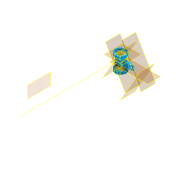
# Autodesk Inventor part: bistability_test_rack_45_0.8
Saved by Autodesk Inventor 2021 (Build 250183000, 183)
## iProperties
Created: 2021-01-14
Part Number: bistability_test_rack_45_0.8
Material: Generic
Document SubType Name: Modeling
Designer: Fierce PC
Density: 1 g/cm^3
Appearance: Default
Author: Fierce PC
Autodesk Inventor part; units mm, degrees
ref_plane "XZ Plane" through (0, 0, 0) normal (0, 1, 0) x (-1, 0, 0)
sketch "Sketch2" plane through (0, 0, 0) normal (0, 1, 0) x (-1, 0, 0)
  circle A0 centre (0, 0) radius 2
  circle A1 centre (0, 0) radius 1
  dimension "d0" = 4
  dimension "d1" = 2
  constraints: 2 centre point, 2 coincident
  measures "d0" diameter of A0
  measures "d1" diameter of A1
extrude "Extrusion1" add sketch "Sketch2" along normal blind 2 and the other way blind 2.5
sketch "Sketch3" plane through (0, 0, 0) normal (1, 0, 0) x (0, 1, 0)
  line L0 (2, -2) -> (2, 2) projected
  line L1 (-4.506, 0) -> (6.036, 0) projected
  line L2 (-2.5, 2) -> (2, 2) projected
  line L3 (-2.5, 4) -> (2, 4) projected
  arc A0 (2.1798, 2.5374) -> (2, 2) centre (2.8929, 2) ccw
  line L4 (2, 2) -> (2, 1)
  line L5 (2, 1) -> (-2.5, 1) projected
  line L6 (2.7766, 1) -> (2, 1)
  line L7 (2.7766, 1) -> (2.7766, 2)
  line L8 (2.7766, 2) -> (4.6605, 4.5)
  line L9 (2.1798, 2.5374) -> (3.6587, 4.5)
  line L10 (4.6605, 4.5) -> (3.6587, 4.5)
  point P0 (0, 0)
  dimension "d95" = 37
  dimension "d96" = 0.8
  dimension "d99" = 2.5
  constraints: 12 end point, 2 horizontal alignment, 2 point on circle, 2 point on line, 2 tangent, 1 centre point, 1 horizontal, 1 parallel, 1 perpendicular, 1 vertical, 1 other
  measures "d96" distance between parallel lines of L8 L9
  measures "d99" vertical distance of L7.end L8.end
revolve "Revolution1" add sketch "Sketch3" angle 360 about axis through (0, -10, 0) along (0, 1, 0) separate body
sketch "Sketch4" plane through (0, 0, 0) normal (0, 0, 1) x (1, 0, 0)
  line L0 (0, -0.906) -> (0, 5.436) projected
  line L1 (4.5, 4.6605) -> (-4.5, 4.6605) projected
  line L2 (4.5, 4.6605) -> (6.5, 4.6605)
  line L3 (6.5, 4.6605) -> (6.5, 3.6587)
  line L4 (6.5, 3.6587) -> (4.5, 3.6587)
  line L5 (4.5, 3.6587) -> (4.5, 4.6605)
  line L6 (2.5374, 2.1798) -> (4.5, 3.6587) projected
  line L7 (4.5, 3.6587) -> (4.5, 4.6605) projected
  point P0 (0, 0)
  dimension "d178" = 2
  constraints: 8 end point, 2 parallel, 1 coincident, 1 horizontal, 1 perpendicular
  measures "d178" distance of L1.start L2.end
revolve "Revolution2" add sketch "Sketch4" angle 360 about axis through (0, -10, 0) along (0, 1, 0) separate body
sketch "Sketch15" plane through (0, -2.5, 0) normal (0, -1, 0) x (1, 0, 0)
  circle A0 centre (0, 0) radius 2.7574 projected
  circle A1 centre (0, 0) radius 2
  dimension "d73" = 4
  constraints: 1 centre point, 1 coincident
  measures "d73" diameter of A1
extrude "Extrusion9" add sketch "Sketch15" along normal blind 0.5 contours A1 bodies 1
ref_plane "Work Plane6" through (0, 0, 0) normal (0.1736482, 0, 0.9848078) x (0, 1, 0)
ref_plane "Work Plane5" through (4.7625, 0, 0) normal (1, 0, 0) x (0, 1, 0)
sketch "Sketch21" plane through (0, 4.6605, 0) normal (0, 1, 0) x (1, 0, 0)
  arc A0 (-3.2392, 7.3149) -> (-5.022, 6.2273) centre (0, 0) ccw
  arc A1 (-3.6238, 8.1836) -> (-5.6184, 6.9668) centre (0, 0) ccw
  line L0 (-5.6184, 6.9668) -> (-5.022, 6.2273)
  line L1 (-3.2392, 7.3149) -> (-3.6238, 8.1836)
  dimension "d100" = 15
  dimension "d101" = 0.95
  constraints: 4 end point, 4 point on circle, 2 centre point, 1 coincident
  measures "d101" radial gap between concentric circles of A0 A1
extrude "Extrusion13" [suppressed]
sketch "Sketch23" plane through (-5.022, 7.0569, -6.2273) normal (-0.778413, 0, 0.6277525) x (0.6277525, 0, 0.778413)
  line L0 (-0.95, 2.3) -> (0, 2.3) projected
  line L1 (0, 0) -> (0, 2.3) projected
  line L2 (-0.95, 2.3) -> (0, 2.3)
  line L3 (0, 2.3) -> (0, 1.1)
  line L4 (0, 1.1) -> (-0.95, 1.1)
  line L5 (-0.95, 1.1) -> (-0.95, 2.3)
  line L6 (8, -14.3283) -> (8, 5.0714) projected
  point P0 (8, -7.0569)
  dimension "d105" = 1.2
  constraints: 8 end point, 2 parallel, 1 horizontal, 1 perpendicular, 1 point on line
  measures "d105" distance between parallel lines of L0 L4
revolve "Revolution3" [suppressed]
fillet "Fillet3" [suppressed]
pattern_circular "Circular Pattern5" [suppressed]
ref_plane "Work Plane8" through (4, 0, 0) normal (1, 0, 0) x (0, 1, 0)
sketch "Sketch26" plane through (4, 0, 0) normal (1, 0, 0) x (0, 1, 0)
  line L0 (-3, 2) -> (-3, -2) projected
  line L1 (0, -4) -> (-3, -4)
  line L2 (-3, -4) -> (-3, 4)
  line L3 (-3, 4) -> (0, 4)
  line L4 (0, 4) -> (0, -4)
  point P0 (0, 0)
  point P1 (0, 0)
  point P2 (-4, -3)
  dimension "d115" = 8
  dimension "d117" = 3
  constraints: 8 end point, 2 parallel, 1 coincident, 1 horizontal, 1 midpoint, 1 perpendicular, 1 point on line
  measures "d115" distance of L3.end L1.start
  measures "d117" distance of L1.start L1.end
extrude "Extrusion14" add sketch "Sketch26" against normal up to surface (4 mm away) bodies 1
pattern_circular "Circular Pattern6" count 2 over 360 about axis through (0, 4.1596, 0) along (0, -1, 0) of "Extrusion14" bodies 1
sketch "Sketch27" plane through (0, 4.6605, 0) normal (0, 1, 0) x (1, 0, 0)
  circle A0 centre (0, 0) radius 2.5374 projected
  circle A1 centre (0, 0) radius 6.5
  circle A2 centre (0, 0) radius 5.5
  dimension "d125" = 1
  dimension "d128" = 13
  constraints: 2 centre point, 2 coincident
  measures "d125" radial gap between concentric circles of A1 A2
  measures "d128" diameter of A1
extrude "Extrusion15" add sketch "Sketch27" along normal blind 2 contours A1 bodies 3
mirror "Mirror3" about plane through (0, -3, 0) normal (0, -1, 0) bodies 3 2 1
sketch "Sketch19" plane through (4.7625, 0, 0) normal (1, 0, 0) x (0, 1, 0)
  line L0 (-1, 3) -> (-7, 3)
  line L1 (-7, 3) -> (-7, 6.2171)
  line L2 (-7, 6.2171) -> (-1, 6.2171)
  line L3 (-1, 6.2171) -> (-1, 3)
  line L4 (-1, -3) -> (-7, -3)
  line L5 (-7, -3) -> (-7, -7.1834)
  line L6 (-7, -7.1834) -> (-1, -7.1834)
  line L7 (-1, -7.1834) -> (-1, -3)
  point P0 (0, 0)
  dimension "d81" = 6
  dimension "d82" = 7
  dimension "d83" = 3
  dimension "d84" = 6
  dimension "d85" = 3
  constraints: 16 end point, 4 parallel, 2 horizontal, 2 perpendicular
  measures "d81" distance of L1.end L2.end
  measures "d82" horizontal distance of L0.end point (0, 0)
  measures "d83" distance from line of point (0, 0) L0
  measures "d84" distance of L5.end L6.end
  measures "d85" distance from line of L4 point (0, 0)
extrude "Extrusion11" [suppressed]
fillet "Fillet2" radius 2 2 edges at (0, 2.7766, -2) (0, -8.7766, -2)
sketch "Sketch34" plane through (0, -6, 0) normal (0, -1, 0) x (1, 0, 0)
  circle A0 centre (0, 0) radius 1
  dimension "d160" = 2
  constraints: 1 centre point, 1 coincident
  measures "d160" diameter of A0
extrude "Extrusion20" cut sketch "Sketch34" against normal blind 1.5 bodies 1
ref_plane "Work Plane15" through (-3, 0, -5) normal (0, 1, 0) x (1, 0, 0)
sketch "Sketch36" plane through (-3, 0, -5) normal (0, 1, 0) x (1, 0, 0)
  circle A0 centre (3, -5) radius 1
  dimension "d161" = 2
  constraints: 1 centre point, 1 coincident
  measures "d161" diameter of A0
extrude "Extrusion22" cut sketch "Sketch36" against normal blind 1.5 bodies 1
ref_plane "Work Plane10" through (-3, -3, -5) normal (0, 1, 0) x (1, 0, 0)
ref_plane "Work Plane12" through (18.7928, 10.85, 0) normal (0.8660254, 0.5, 0) x (0, 0, 1)
ref_plane "Work Plane11" through (0, 0, 0) normal (0.8660254, 0.5, 0) x (0, 0, 1)
ref_plane "Work Plane14" through (21.3908, -12.35, 0) normal (0.8660254, -0.5, 0) x (0, 0, 1)
ref_plane "Work Plane13" through (0, 0, 0) normal (0.8660254, -0.5, 0) x (0, 0, 1)
sketch "Sketch39" plane through (4, 0, 0) normal (1, 0, 0) x (0, 0, -1)
  line L0 (-4, 0) -> (4, 0) projected
  line L1 (4, 0) -> (4, -6) projected
  line L2 (4, -6) -> (-4, -6) projected
  line L3 (-4, -6) -> (-4, 0) projected
  line L4 (-2.0616, 3.6587) -> (-2.0616, 4.6605) projected
  line L5 (2.0616, 4.6605) -> (2.0616, 3.6587) projected
  line L6 (2.0616, -9.6587) -> (2.0616, -10.6605) projected
  line L7 (-2.0616, -10.6605) -> (-2.0616, -9.6587) projected
  line L8 (-2.0616, 4.6605) -> (-2.0616, 3.6587) projected
  line L9 (-2.0616, 3.6587) -> (-5.1235, 3.6587) projected
  line L10 (-5.1235, 3.6587) -> (-5.1235, 6.6605) projected
  line L11 (-5.1235, 6.6605) -> (-3.7749, 6.6605) projected
  line L12 (-3.7749, 6.6605) -> (-3.7749, 4.6605) projected
  line L13 (-3.7749, 4.6605) -> (-2.0616, 4.6605) projected
  line L14 (2.0616, 3.6587) -> (2.0616, 4.6605) projected
  line L15 (2.0616, 4.6605) -> (3.7749, 4.6605) projected
  line L16 (3.7749, 4.6605) -> (3.7749, 6.6605) projected
  line L17 (3.7749, 6.6605) -> (5.1235, 6.6605) projected
  line L18 (5.1235, 6.6605) -> (5.1235, 3.6587) projected
  line L19 (5.1235, 3.6587) -> (2.0616, 3.6587) projected
  line L20 (-2.0616, -9.6587) -> (-2.0616, -10.6605) projected
  line L21 (-2.0616, -10.6605) -> (-3.7749, -10.6605) projected
  line L22 (-3.7749, -10.6605) -> (-3.7749, -12.6605) projected
  line L23 (-3.7749, -12.6605) -> (-5.1235, -12.6605) projected
  line L24 (-5.1235, -12.6605) -> (-5.1235, -9.6587) projected
  line L25 (-5.1235, -9.6587) -> (-2.0616, -9.6587) projected
  line L26 (2.0616, -10.6605) -> (2.0616, -9.6587) projected
  line L27 (2.0616, -9.6587) -> (5.1235, -9.6587) projected
  line L28 (5.1235, -9.6587) -> (5.1235, -12.6605) projected
  line L29 (5.1235, -12.6605) -> (3.7749, -12.6605) projected
  line L30 (3.7749, -12.6605) -> (3.7749, -10.6605) projected
  line L31 (3.7749, -10.6605) -> (2.0616, -10.6605) projected
  point P0 (0, 0)
  point P1 (-0.37, -3)
  point P2 (0.37, -3)
  constraints: 4 horizontal alignment
sketch "Sketch40" plane through (4, 0, 0) normal (1, 0, 0) x (0, 0, -1)
  circle A0 centre (0, -1.3621) radius 0.5 projected
  point P0 (0, 0)
sketch "Sketch41" plane through (4, 0, 0) normal (1, 0, 0) x (0, 0, -1)
  line L0 (4, -6) -> (-4, -6) projected
  line L1 (4, 0) -> (-4, 0) projected
  line L2 (-4, 0) -> (-4, -6) projected
  line L3 (4, -6) -> (-4, -6) projected
  line L4 (4, -6) -> (4, 0) projected
  line L5 (4, -6) -> (4, 0) projected
  arc A0 (4, -4.5) -> (2.5, -6) centre (4, -6) ccw
  line L6 (4, 0) -> (-4, 0) projected
  arc A1 (2.5, 0) -> (4, -1.5) centre (4, 0) ccw
  arc A2 (-4, -1.5) -> (-2.5, 0) centre (-4, 0) ccw
  line L7 (-4, 0) -> (-4, -6) projected
  arc A3 (-2.5, -6) -> (-4, -4.5) centre (-4, -6) ccw
  point P0 (0, 0)
  point P1 (-4, -6)
  point P2 (-2.5, 0)
  dimension "d181" = 1.5
  constraints: 8 point on circle, 4 centre point, 4 coincident, 4 point on line, 3 equal radius
  measures "d181" radius of A0
extrude "Extrusion25" cut sketch "Sketch41" against normal up to next contours L0 A0 L4 | L0 L2 A3 | A1 L1 L4 | L2 L1 A2 bodies 1
sketch "Sketch43" plane through (4, 0, 0) normal (1, 0, 0) x (0, 0, -1)
  line L0 (2, 0) -> (-2, 0) projected
  line L1 (-2.5, -6) -> (2.5, -6) projected
  line L2 (-1.3, 0) -> (1.3, 0)
  line L3 (1.3, 0) -> (1.3, -6)
  line L4 (1.3, -6) -> (-1.3, -6)
  line L5 (-1.3, -6) -> (-1.3, 0)
  arc A0 (4, -4.5) -> (2.5, -6) centre (4, -6) ccw projected
  line L6 (2.5, -6) -> (-2.5, -6) projected
  arc A1 (-2.5, -6) -> (-4, -4.5) centre (-4, -6) ccw projected
  line L7 (-4, -4.5) -> (-4, -1.5) projected
  arc A2 (-4, -1.5) -> (-2.5, 0) centre (-4, 0) ccw projected
  line L8 (-2.5, 0) -> (2.5, 0) projected
  arc A3 (2.5, 0) -> (4, -1.5) centre (4, 0) ccw projected
  line L9 (4, -1.5) -> (4, -4.5) projected
  line L10 (-2.0616, 3.6587) -> (-2.0616, 4.6605) projected
  line L11 (2.0616, 4.6605) -> (2.0616, 3.6587) projected
  line L12 (2.0616, -9.6587) -> (2.0616, -10.6605) projected
  line L13 (-2.0616, -10.6605) -> (-2.0616, -9.6587) projected
  line L14 (-2.0616, 4.6605) -> (-2.0616, 3.6587) projected
  line L15 (-2.0616, 3.6587) -> (-5.1235, 3.6587) projected
  line L16 (-5.1235, 3.6587) -> (-5.1235, 6.6605) projected
  line L17 (-5.1235, 6.6605) -> (-3.7749, 6.6605) projected
  line L18 (-3.7749, 6.6605) -> (-3.7749, 4.6605) projected
  line L19 (-3.7749, 4.6605) -> (-2.0616, 4.6605) projected
  line L20 (2.0616, 3.6587) -> (2.0616, 4.6605) projected
  line L21 (2.0616, 4.6605) -> (3.7749, 4.6605) projected
  line L22 (3.7749, 4.6605) -> (3.7749, 6.6605) projected
  line L23 (3.7749, 6.6605) -> (5.1235, 6.6605) projected
  line L24 (5.1235, 6.6605) -> (5.1235, 3.6587) projected
  line L25 (5.1235, 3.6587) -> (2.0616, 3.6587) projected
  line L26 (-2.0616, -9.6587) -> (-2.0616, -10.6605) projected
  line L27 (-2.0616, -10.6605) -> (-3.7749, -10.6605) projected
  line L28 (-3.7749, -10.6605) -> (-3.7749, -12.6605) projected
  line L29 (-3.7749, -12.6605) -> (-5.1235, -12.6605) projected
  line L30 (-5.1235, -12.6605) -> (-5.1235, -9.6587) projected
  line L31 (-5.1235, -9.6587) -> (-2.0616, -9.6587) projected
  line L32 (2.0616, -10.6605) -> (2.0616, -9.6587) projected
  line L33 (2.0616, -9.6587) -> (5.1235, -9.6587) projected
  line L34 (5.1235, -9.6587) -> (5.1235, -12.6605) projected
  line L35 (5.1235, -12.6605) -> (3.7749, -12.6605) projected
  line L36 (3.7749, -12.6605) -> (3.7749, -10.6605) projected
  line L37 (3.7749, -10.6605) -> (2.0616, -10.6605) projected
  point P0 (0, 0)
  point P1 (1.3, 0)
  dimension "d191" = 2.6
  dimension "d192" = 1.3
  constraints: 8 end point, 4 horizontal alignment, 2 parallel, 2 point on line, 1 horizontal, 1 perpendicular
  measures "d191" distance between parallel lines of L3 L5
  measures "d192" distance from line of point (0, 0) L5
extrude "Extrusion26" add sketch "Sketch43" along normal blind 7 contours L3 L1 L5 L0 bodies 1
sketch "Sketch44" plane through (0, 0, 0) normal (0, 0, 1) x (1, 0, 0)
  line L0 (11, -0.5) -> (12.8, -0.5)
  line L1 (12.8, -0.5) -> (12.8, -0.3)
  line L2 (12.8, -0.3) -> (16.3, -0.7)
  line L3 (16.3, -0.7) -> (16.3, -0.9)
  line L4 (16.3, -0.9) -> (11, -0.9)
  line L5 (11, -6) -> (11, 0) projected
  line L6 (11, -1.4) -> (16.9091, -1.4)
  line L7 (-11.1818, -3) -> (21.5909, -3) projected
  point P0 (0, 0)
  dimension "d195" = 1.6
  dimension "d196" = 1
  dimension "d197" = 1.8
  dimension "d198" = 1.4
  dimension "d199" = 2.2
  dimension "d200" = 3.5
  dimension "d201" = 1.8
  constraints: 12 end point, 2 horizontal, 2 perpendicular, 2 point on line, 1 parallel, 1 vertical alignment
  measures "d195" distance between parallel lines of L7 L6
  measures "d196" diameter of L4 L6
  measures "d197" diameter of L0 L6
  measures "d198" diameter of L2.end L6
  measures "d199" diameter of L1.end L6
  measures "d200" distance between parallel lines of L1 L3
  measures "d201" distance of L0.start L0.end
revolve "Revolution5" add sketch "Sketch44" angle 360 about axis through (11, -1.4, 0) along (1, 0, 0) bodies 1
sketch "Sketch45" plane through (11, -1.4, 0) normal (1, 0, 0) x (0, 0, -1)
  circle A0 centre (0, 0) radius 0.5
  point P0 (0, 1.4)
  constraints: 1 centre point
extrude "Extrusion27" cut sketch "Sketch45" against normal up to surface (11 mm away) bodies 1
mirror "Mirror12" about plane through (-3, -3, -5) normal (0, 1, 0) of "Revolution5", "Extrusion27" bodies 1
body "Solid1"
body "Solid2"
body "Solid3"
